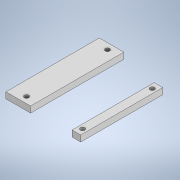
# Autodesk Inventor part: 1111111
Saved by Autodesk Inventor 2020 (Build 240168000, 168)
## iProperties
Created: 2022-11-21
Part Number: 1111111
Material: Типовые
Document SubType Name: Modeling
Designer: TRENER
Density: 1 g/cm^3
Appearance: По умолчанию
Author: TRENER
Autodesk Inventor part; units mm, degrees
ref_plane "YZ Plane" through (0, 0, 0) normal (1, 0, 0) x (0, 1, 0)
ref_plane "XZ Plane" through (0, 0, 0) normal (0, 1, 0) x (-1, 0, 0)
ref_plane "XY Plane" through (0, 0, 0) normal (0, 0, 1) x (1, 0, 0)
sketch "Эскиз1" plane through (0, 0, 0) normal (0, 1, 0) x (-1, 0, 0)
  line L0 (12.3801, 21.759) -> (0.3801, 21.759)
  line L1 (0.3801, 21.759) -> (0.3801, -23.741)
  line L2 (0.3801, -23.741) -> (12.3801, -23.741)
  line L3 (12.3801, -23.741) -> (12.3801, 21.759)
  line L4 (-24.0729, 21.759) -> (-19.8729, 21.759)
  line L5 (-19.8729, 21.759) -> (-19.8729, -18.241)
  line L6 (-19.8729, -18.241) -> (-24.0729, -18.241)
  line L7 (-24.0729, -18.241) -> (-24.0729, 21.759)
  line L8 (5.3801, 21.759) -> (5.3801, 18.759) construction
  line L9 (5.3801, -23.741) -> (5.3801, -20.741) construction
  line L10 (-21.9729, -18.241) -> (-21.9729, -15.241) construction
  line L11 (-21.9729, 21.759) -> (-21.9729, 18.759) construction
  circle A0 centre (-21.9729, 18.759) radius 1.1
  circle A1 centre (-21.9729, -15.241) radius 1.1
  circle A2 centre (5.3801, 18.759) radius 1.1
  circle A3 centre (5.3801, -20.741) radius 1.1
  point P0 (0, 0)
  dimension "d0" = 45.5
  dimension "d1" = 12
  dimension "d20" = 4.2
  dimension "d21" = 40
  dimension "d22" = 3
  dimension "d23" = 3
  dimension "d24" = 3
  dimension "d25" = 3
  dimension "d26" = 2.2
  dimension "d27" = 2.2
  dimension "d28" = 2.2
  dimension "d29" = 2.2
  dimension "d30" = 5
  dimension "d31" = 5
  constraints: 24 end point, 4 centre point, 4 coincident, 4 parallel, 4 vertical, 2 horizontal, 2 midpoint, 2 perpendicular, 2 point on line
  measures "d0" distance of L2.end L0.start
  measures "d1" distance of L1.end L2.end
  measures "d20" distance of L4.start L4.end
  measures "d21" distance of L6.end L4.start
  measures "d22" distance of L8.start L8.end
  measures "d23" distance of L9.start L9.end
  measures "d24" distance of L10.start L10.end
  measures "d25" distance of L11.start L11.end
  measures "d26" diameter of A0
  measures "d27" diameter of A1
  measures "d28" diameter of A2
  measures "d29" diameter of A3
  measures "d30" distance from line of L1 A2.centre
  measures "d31" distance from line of L1 A3.centre
extrude "Выдавливание1" add sketch "Эскиз1" along normal blind 3
